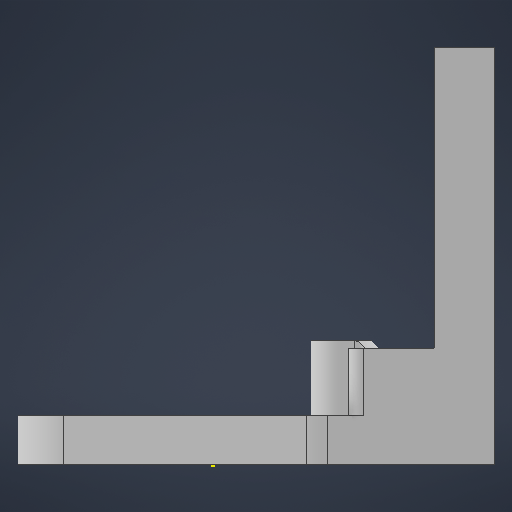
# Autodesk Inventor part: guideline
Saved by Autodesk Inventor 2026 (Build 300175000, 175)
## iProperties
Created: 2025-11-28
Part Number: guideline
Material: 一般
Document SubType Name: Modeling
Designer: numai
Density: 1 g/cm^3
Appearance: 既定
Author: numai
Autodesk Inventor part; units mm, degrees
ref_plane "YZ Plane" through (0, 0, 0) normal (1, 0, 0) x (0, 1, 0)
ref_plane "XZ Plane" through (0, 0, 0) normal (0, 1, 0) x (-1, 0, 0)
ref_plane "XY Plane" through (0, 0, 0) normal (0, 0, 1) x (1, 0, 0)
sketch "スケッチ1" plane through (0, 0, 0) normal (0, 0, 1) x (1, 0, 0)
  circle A0 centre (0, 0) radius 17 construction
  line L0 (0, 0) -> (0, 20.4) construction
  circle A1 centre (0, -17) radius 3 construction
  circle A2 centre (0, 0) radius 14 construction
  circle A3 centre (0, 0) radius 20 construction
  circle A4 centre (0, 17) radius 3 construction
  circle A5 centre (-8.5, 14.7224) radius 3 construction
  line L1 (-8.5, 14.7224) -> (0, 17) construction
  line L2 (-8.5, 14.7224) -> (0, 0) construction
  line L3 (-8.5, 14.7224) -> (8.5, 14.7224) construction
  line L4 (0, 0) -> (8.5, 14.7224) construction
  line L5 (0, 17) -> (8.5, 14.7224) construction
  circle A6 centre (8.5, 14.7224) radius 3 construction
  arc A7 (-32.8415, 8.2002) -> (32.8415, 8.2002) centre (0, 17) ccw construction
  line L6 (-8.5, 14.7224) -> (-32.8415, 8.2002) construction
  line L7 (8.5, 14.7224) -> (32.8415, 8.2002) construction
  arc A8 (-8.5, 14.7224) -> (8.5, 14.7224) centre (0, 17) ccw construction
  circle A9 centre (0, 8.2002) radius 3 construction
  line L8 (3, 8.2002) -> (3, -17) construction
  line L9 (-3, 8.2002) -> (-3, -17) construction
  circle A10 centre (0, -17) radius 9 construction
  line L10 (0, -20) -> (0, -26) construction
  circle A11 centre (0, 17) radius 9 construction
  circle A12 centre (0, 17) radius 7 construction
  line L11 (-4.9497, 21.9497) -> (4.9497, 21.9497) construction
  line L12 (4.9497, 21.9497) -> (4.9497, 12.0503) construction
  line L13 (4.9497, 12.0503) -> (-4.9497, 12.0503) construction
  line L14 (-4.9497, 12.0503) -> (-4.9497, 21.9497) construction
  circle A13 centre (0, 17) radius 2.5
  line L15 (0, 8.2002) -> (0, -17) construction
  line L16 (-3, 8.2002) -> (-3, -17)
  line L17 (3, -17) -> (3, 8.2002)
  arc A14 (3, 8.2002) -> (-3, 8.2002) centre (0, 8.2002) ccw
  arc A15 (-3, -17) -> (3, -17) centre (0, -17) ccw
  line L18 (0, 17) -> (0, -17) construction
  line L19 (-9, 17) -> (-9, -17)
  line L20 (9, -17) -> (9, 17)
  arc A16 (9, 17) -> (-9, 17) centre (0, 17) ccw
  arc A17 (-9, -17) -> (9, -17) centre (0, -17) ccw
  circle A18 centre (4.9497, 21.9497) radius 1.25
  circle A19 centre (-4.9497, 21.9497) radius 1.25
  circle A20 centre (-4.9497, 12.0503) radius 1.25
  circle A21 centre (4.9497, 12.0503) radius 1.25
  circle A22 centre (0, 17) radius 20 construction
  circle A23 centre (0, -17) radius 34 construction
  circle A24 centre (-10.8551, 15.2206) radius 9 construction
  circle A25 centre (10.8551, 15.2206) radius 9 construction
  line L21 (-19.3841, 12.3472) -> (-8.529, -19.8734)
  line L22 (19.3841, 12.3472) -> (8.529, -19.8734)
  arc A26 (13.7285, 23.7496) -> (-13.7285, 23.7496) centre (0, -17) ccw construction
  arc A27 (-13.7285, 23.7496) -> (-19.3841, 12.3472) centre (-10.8551, 15.2206) ccw construction
  arc A28 (19.3841, 12.3472) -> (13.7285, 23.7496) centre (10.8551, 15.2206) ccw construction
  line L23 (19.8551, 37.35) -> (-19.8551, 37.35)
  line L24 (19.8551, 37.35) -> (19.8551, 15.2206)
  line L25 (-19.8551, 37.35) -> (-19.8551, 15.2206)
  arc A29 (19.3841, 12.3472) -> (19.8551, 15.2206) centre (10.8551, 15.2206) ccw
  arc A30 (-19.8551, 15.2206) -> (-19.3841, 12.3472) centre (-10.8551, 15.2206) ccw
  line L26 (19.8551, 29.35) -> (-19.8551, 29.35) construction
  line L27 (19.8551, 33.35) -> (-19.8551, 33.35) construction
  line L28 (-15.8551, 29.35) -> (-15.8551, 37.35) construction
  line L29 (15.8551, 29.35) -> (15.8551, 37.35) construction
  circle A31 centre (15.8551, 33.35) radius 1.25
  circle A32 centre (0, 33.35) radius 1.25
  circle A33 centre (-15.8551, 33.35) radius 1.25
  point P0 (-5.6022, 15.4989)
  point P1 (-2.8978, 16.2235)
  point P2 (0, -4.3999)
  point P3 (0, 26)
  point P4 (0, 10.2)
  dimension "d7" = 18
  dimension "d0" = 34
  dimension "d2" = 6
  dimension "d4" = 2.7999
  dimension "d5" = 150
  dimension "d6" = 6
  dimension "d8" = 14
  dimension "d11" = 5
  dimension "d14" = 2.5
  dimension "d15" = 17
  dimension "d16" = 40
  dimension "d17" = 10.2
  dimension "d18" = 20.35
  dimension "d19" = 8
  dimension "d20" = 4
  dimension "d21" = 4
  dimension "d22" = 4
  dimension "d23" = 2.5
  constraints: 64 end point, 45 point on circle, 29 centre point, 22 coincident, 17 tangent, 13 point on line, 7 equal radius, 6 midpoint, 6 vertical, 5 horizontal, 5 perpendicular, 4 parallel, 3 vertical alignment, 1 concentric, 24 other
  measures "d0" diameter of A0
  measures "d2" diameter of A1
  measures "d4" distance of point (-5.602, 15.499) point (-2.898, 16.224)
  measures "d5" angle of L5 L1
  measures "d6" distance of L10.start L10.end
  measures "d8" diameter of A12
  measures "d11" diameter of A13
  measures "d14" diameter of A18
  measures "d15" distance of L1.end point (0, 0)
  measures "d16" diameter of A22
  measures "d17" distance of point (0, 10.2) point (0, 0)
  measures "d18" distance from line of L23 L1.end
  measures "d19" distance between parallel lines of L23 L26
  measures "d20" distance between parallel lines of L23 L27
  measures "d21" distance between parallel lines of L25 L28
  measures "d22" distance between parallel lines of L29 L24
  measures "d23" diameter of A31
extrude "押し出し1" add sketch "スケッチ1" along normal blind 6.5
sketch "スケッチ2" plane through (0, 0, 6.5) normal (0, 0, 1) x (1, 0, 0)
  arc A0 (-8.529, -19.8734) -> (8.529, -19.8734) centre (0, -17) ccw projected
  line L0 (8.529, -19.8734) -> (19.3841, 12.3472) projected
  arc A1 (19.3841, 12.3472) -> (19.8551, 15.2206) centre (10.8551, 15.2206) ccw projected
  line L1 (19.8551, 15.2206) -> (19.8551, 37.35) projected
  line L2 (19.8551, 37.35) -> (-19.8551, 37.35) projected
  line L3 (-19.8551, 37.35) -> (-19.8551, 15.2206) projected
  arc A2 (-19.8551, 15.2206) -> (-19.3841, 12.3472) centre (-10.8551, 15.2206) ccw projected
  line L4 (-19.3841, 12.3472) -> (-8.529, -19.8734) projected
  circle A3 centre (-4.9497, 12.0503) radius 1.25 projected
  circle A4 centre (4.9497, 12.0503) radius 1.25 projected
  circle A5 centre (-4.9497, 21.9497) radius 1.25 projected
  circle A6 centre (4.9497, 21.9497) radius 1.25 projected
  arc A7 (3, 8.2002) -> (-3, 8.2002) centre (0, 8.2002) ccw projected
  line L5 (3, 8.2002) -> (3, -17) projected
  arc A8 (-3, -17) -> (3, -17) centre (0, -17) ccw projected
  line L6 (-3, -17) -> (-3, 8.2002) projected
  circle A9 centre (0, 17) radius 2.5 projected
  circle A10 centre (-15.8551, 33.35) radius 1.25 projected
  circle A11 centre (0, 33.35) radius 1.25 projected
  circle A12 centre (15.8551, 33.35) radius 1.25 projected
  circle A13 centre (0, 17) radius 10
  circle A14 centre (0, 17) radius 4
  line L7 (0, 17) -> (0.6946, 20.9392) construction
  line L8 (0.6946, 20.9392) -> (9.7205, 19.3477)
  line L9 (0, 17) -> (0, 37.35) construction
  arc A15 (4.6338, 20.2446) -> (3.5681, 18.8079) centre (4.4602, 19.2598) ccw
  line L10 (0, 17) -> (-0.6946, 20.9392) construction
  line L11 (-0.6946, 20.9392) -> (-9.7933, 19.3349)
  arc A16 (-3.5681, 18.8079) -> (-4.6338, 20.2446) centre (-4.4602, 19.2598) ccw
  line L12 (19.8551, 29.35) -> (-19.8551, 29.35)
  line L13 (-9.7933, 19.3349) -> (-19.8551, 17.5607)
  line L14 (9.7205, 19.3477) -> (19.8551, 17.5607)
  point P0 (0, 0)
  point P1 (-9.7205, 19.3477)
  dimension "d24" = 20
  dimension "d25" = 8
  dimension "d26" = 10
  dimension "d27" = 1
  dimension "d28" = 10
  dimension "d29" = 8
  constraints: 16 end point, 8 point on circle, 6 point on line, 5 tangent, 3 centre point, 2 coincident, 2 collinear, 1 equal radius, 1 midpoint, 1 parallel, 1 perpendicular, 3 other
  measures "d25" diameter of A14
  measures "d26" angle of L9 L7
  measures "d27" radius of A15
  measures "d28" angle of L10 L9
  measures "d29" distance between parallel lines of L12 L2
extrude "押し出し2" add sketch "スケッチ2" along normal blind 10 contours L3 L12 L1 L14 A13 L11 L13 | L8 A14 L11 A13 | A15 A14 L8 | L11 A14 A16 | A14
sketch "スケッチ3" plane through (0, 0, 16.5) normal (0, 0, 1) x (1, 0, 0)
  line L0 (-19.8551, 17.5607) -> (-4.6338, 20.2446) projected
  arc A0 (-3.5681, 18.8079) -> (-4.6338, 20.2446) centre (-4.4602, 19.2598) ccw projected
  arc A1 (-3.5681, 18.8079) -> (3.5681, 18.8079) centre (0, 17) ccw projected
  arc A2 (4.6338, 20.2446) -> (3.5681, 18.8079) centre (4.4602, 19.2598) ccw projected
  line L1 (4.6338, 20.2446) -> (19.8551, 17.5607) projected
  circle A3 centre (0, 17) radius 2.5 projected
  circle A4 centre (-4.9497, 21.9497) radius 1.25 projected
  circle A5 centre (4.9497, 21.9497) radius 1.25 projected
  arc A6 (3.5681, 18.8079) -> (-3.5681, 18.8079) centre (0, 17) ccw
  line L2 (19.8551, 17.5607) -> (19.8551, 29.35) projected
  line L3 (19.8551, 29.35) -> (-19.8551, 29.35) projected
  line L4 (-19.8551, 29.35) -> (-19.8551, 17.5607) projected
  point P0 (0, 0)
  constraints: 2 point on circle, 1 centre point, 1 coincident
extrude "押し出し3" cut sketch "スケッチ3" against normal blind 1 contours L4 L3 L2 L1 A2 A6 A0 L0
sketch "スケッチ4" plane through (0, 0, 6.5) normal (0, 0, 1) x (1, 0, 0)
  line L0 (-19.8551, 29.35) -> (19.8551, 29.35) projected
  line L1 (19.8551, 29.35) -> (19.8551, 37.35) projected
  line L2 (19.8551, 37.35) -> (-19.8551, 37.35) projected
  line L3 (-19.8551, 37.35) -> (-19.8551, 29.35) projected
  circle A0 centre (-15.8551, 33.35) radius 1.25 projected
  circle A1 centre (0, 33.35) radius 1.25 projected
  circle A2 centre (15.8551, 33.35) radius 1.25 projected
  point P0 (0, 0)
extrude "押し出し4" add sketch "スケッチ4" along normal blind 49
sketch "スケッチ5" plane through (0, 0, 0) normal (0, 0, -1) x (-1, 0, 0)
  point P0 (0, 0)
chamfer "面取り1" distance 1 angle 45 1 edges at (0, 21, 15.5)
fillet "フィレット1" radius 2 2 edges at (-19.8551, 17.5607, 11) (19.8551, 17.5607, 11)
equation "\"d20\" = 0.5 * d19"
equation "\"d21\" = d20"
equation "\"d22\" = d21"
equation "\"d28\" = d26"
